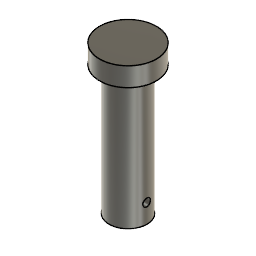
knuckle_joint_assembly (Autodesk Fusion 360 archive; units mm, degrees)
design "pin-knuckle_joint"
part number: 2026-03-14-10-57-53-012
Autodesk Fusion 360 part; units mm, degrees
sketch "Sketch1" plane through (0, 0, 0) normal (0, 0, 1) x (1, 0, 0)
  circle A0 centre (0, 0) radius 22.5
  dimension "d1" = 45
  constraint coincident A0.centre origin
  measures "d1" diameter of A0
extrude "Extrude1" add sketch "Sketch1" against normal blind 15
sketch "Sketch2" plane through (0, 0, -15) normal (0, 0, -1) x (1, 0, 0)
  circle A0 centre (0, 0) radius 22.5
  circle A1 centre (0, 0) radius 15
  dimension "d4" = 30
  constraint coincident A0.centre A1.centre
  measures "d4" diameter of A1
extrude "Extrude2" add sketch "Sketch2" along normal blind 102 contours A1
ref_plane "WorkPlane1" through (-15, 0, 0) normal (1, 0, 0) x (0, 1, 0)
sketch "Sketch5" plane through (-15, 0, 0) normal (1, 0, 0) x (0, 1, 0)
  line L0 (-15, -117) -> (15, -117)
  circle A0 centre (0, -102) radius 3
  dimension "d9" = 6
  measures "d9" diameter of A0
extrude "Extrude3" cut sketch "Sketch5" along normal blind 36

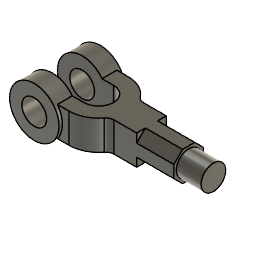
design "fork_sketch"
part number: 2026-03-12-15-10-26-439
Autodesk Fusion 360 part; units mm, degrees
sketch "Sketch7" plane through (0, 0, 0) normal (0, 0, 1) x (1, 0, 0)
  line L0 (31.1769, 18) -> (109, 18)
  line L1 (109, 18) -> (109, -18)
  line L2 (109, -18) -> (31.1769, -18)
  line L3 (0, 0) -> (123.9177, 0)
  line L4 (0, 36) -> (-38, 36)
  line L5 (0, -36) -> (-38, -36)
  line L6 (-38, 36) -> (-38, 18)
  line L7 (-38, -36) -> (-38, -18)
  arc A0 (31.1769, 18) -> (0, 36) centre (0, 0) ccw
  arc A1 (0, -36) -> (31.1769, -18) centre (0, 0) ccw
  arc A2 (0, -18) -> (0, 18) centre (0, 0) ccw
  line L8 (-38, 18) -> (0, 18)
  line L9 (-38, -18) -> (0, -18)
  dimension "d16" = 36
  dimension "d17" = 109
  dimension "d18" = 38
  dimension "d19" = 18
  dimension "d21" = 36
  dimension "d22" = 36
  constraint coincident L3.start A0.centre
  constraint concentric A1 A2
  constraint horizontal L0
  constraint vertical L1
  constraint horizontal L2
  constraint perpendicular L1 L3
  constraint symmetric L0 L2 L3
  constraint tangent L4 A0
  constraint symmetric L3 L4.start L5.start
  constraint symmetric L3 L4.end L5.end
  constraint perpendicular L4 L6
  constraint symmetric L3 L6.end L7.end
  constraint concentric A0 A1
  constraint tangent A2 L8
  constraint tangent A2 L9
  measures "d16" distance of L0.end L1.end
  measures "d17" distance of L3.start L1
  measures "d18" distance of L4.start L4.end
  measures "d19" distance of L4.end L6.end
  measures "d21" diameter of A2
  measures "d22" radius of A0
extrude "Extrude3" add sketch "Sketch7" along normal blind 36
sketch "Sketch8" plane through (0, -18, 0) normal (0, 1, 0) x (-1, 0, 0)
  line L0 (0, 0) -> (38, 0)
  line L1 (38, 0) -> (38, 36)
  line L2 (38, 36) -> (0, 36)
  line L3 (0, 36) -> (0, 0)
  circle A0 centre (38, 18) radius 30
  circle A1 centre (38, 18) radius 15
  dimension "d25" = 60
  dimension "d26" = 30
  constraint midpoint L1 A0.centre
  constraint concentric A0 A1
  measures "d25" diameter of A0
  measures "d26" diameter of A1
extrude "Extrude4" add sketch "Sketch8" against normal blind 22 contours L0 L1 L2 A0 A1 | L0 L1 L2 A0 A1
extrude "Extrude5" cut sketch "Sketch8" against normal blind 40 contours L1 A1 picked at (32.9644, 22.2975)
sketch "Sketch9" plane through (0, 18, 0) normal (0, -1, 0) x (1, 0, 0)
  line L0 (-38, 0) -> (0, 0)
  line L1 (0, 0) -> (0, 36)
  line L2 (0, 36) -> (-38, 36)
  line L3 (-38, 36) -> (-38, 0)
  circle A0 centre (-38, 18) radius 30
  circle A1 centre (-38, 18) radius 15
  dimension "d31" = 60
  dimension "d32" = 30
  constraint midpoint L3 A0.centre
  constraint concentric A0 A1
  measures "d31" diameter of A0
  measures "d32" diameter of A1
extrude "Extrude6" add sketch "Sketch9" against normal blind 22 contours L0 L2 L3 A0 A1 | L0 L2 L3 A0 A1
extrude "Extrude7" cut sketch "Sketch9" against normal blind 26 contours L3 A1 picked at (-35.2114, 22.5991)
sketch "Sketch10" plane through (109, 0, 0) normal (1, 0, 0) x (0, 1, 0)
  line L0 (-18, 0) -> (18, 0)
  line L1 (18, 0) -> (18, 36)
  line L2 (18, 36) -> (-18, 36)
  line L3 (-18, 36) -> (-18, 0)
  line L4 (0, 0) -> (0, 36) construction
  line L5 (-18, 18) -> (18, 18) construction
  line L6 (18, 25.4558) -> (7.4558, 36)
  line L7 (7.4558, 36) -> (-7.4558, 36)
  line L8 (-7.4558, 36) -> (-18, 25.4558)
  line L9 (-18, 25.4558) -> (-18, 10.5442)
  line L10 (-18, 10.5442) -> (-7.4558, 0)
  line L11 (-7.4558, 0) -> (7.4558, 0)
  line L12 (7.4558, 0) -> (18, 10.5442)
  line L13 (18, 10.5442) -> (18, 25.4558)
  point P0 (0, 18)
  constraint coincident L4.start origin
  constraint midpoint L2 L4.end
  constraint midpoint L3 L5.start
  constraint midpoint L1 L5.end
  constraint midpoint L4 P0
extrude "Extrude8" cut sketch "Sketch10" against normal blind 45 contours L1 L2 L6
extrude "Extrude9" cut sketch "Sketch10" against normal blind 45 contours L2 L3 L8
extrude "Extrude10" cut sketch "Sketch10" against normal blind 45 contours L0 L3 L10
extrude "Extrude11" cut sketch "Sketch10" against normal blind 45 contours L0 L1 L12
sketch "Sketch11" plane through (109, 0, 0) normal (1, 0, 0) x (0, 1, 0)
  line L0 (7.4558, 0) -> (18, 10.5442)
  line L1 (18, 10.5442) -> (18, 25.4558)
  line L2 (18, 25.4558) -> (7.4558, 36)
  line L3 (7.4558, 36) -> (-7.4558, 36)
  line L4 (-7.4558, 36) -> (-18, 25.4558)
  line L5 (-18, 25.4558) -> (-18, 10.5442)
  line L6 (-18, 10.5442) -> (-7.4558, 0)
  line L7 (-7.4558, 0) -> (7.4558, 0)
  circle A0 centre (0, 18) radius 15
  dimension "d45" = 30
  measures "d45" diameter of A0
extrude "Extrude12" add sketch "Sketch11" along normal blind 30 contours A0
fillet "Fillet1" radius 10 2 edges at (31.1769, 18, 18) (31.1769, -18, 18)

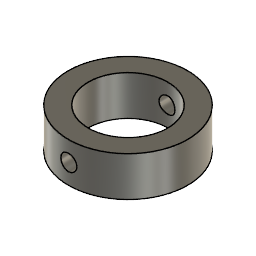
design "COLLAR"
part number: 2026-03-14-12-37-12-628
Autodesk Fusion 360 part; units mm, degrees
sketch "Sketch1" plane through (0, 0, 0) normal (0, 0, 1) x (1, 0, 0)
  circle A0 centre (0, 0) radius 15
  circle A1 centre (0, 0) radius 22.5
  dimension "d1" = 30
  dimension "d2" = 45
  constraint coincident A0.centre A1.centre
  constraint concentric A0 A1
  measures "d1" diameter of A0
  measures "d2" diameter of A1
extrude "Extrude1" add sketch "Sketch1" along normal blind 15
sketch "Sketch2" plane through (0, 0, 0) normal (0, 1, 0) x (1, 0, 0)
ref_plane "WorkPlane1" through (0, -22.5, 0) normal (0, 1, 0) x (0, 0, 1)
sketch "Sketch3" plane through (0, -22.5, 0) normal (0, 1, 0) x (1, 0, 0)
  line L0 (0, 0) -> (0, -15)
  line L1 (-22.5, -15) -> (22.5, -15)
  circle A0 centre (0, -7.5) radius 3
  dimension "d6" = 6
  constraint coincident L0.start origin
  constraint vertical L0
  constraint coincident L0.end L1
  constraint midpoint L0 A0.centre
  measures "d6" diameter of A0
extrude "Extrude2" cut sketch "Sketch3" along normal blind 88

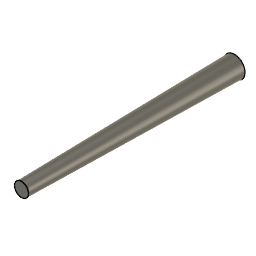
design "taper_pin"
part number: 2026-03-14-12-44-22-029
Autodesk Fusion 360 part; units mm, degrees
sketch "Sketch1" plane through (0, 0, 0) normal (0, 1, 0) x (1, 0, 0)
  circle A0 centre (0, 0) radius 2
  dimension "d1" = 4
  constraint coincident A0.centre origin
  measures "d1" diameter of A0
sketch "Sketch2" plane through (0, 0, 0) normal (0, 1, 0) x (1, 0, 0)
  circle A0 centre (0, 0) radius 2
  dimension "d4" = 4
  constraint coincident A0.centre origin
  measures "d4" diameter of A0
extrude "Extrude2" add sketch "Sketch2" along normal blind 60 draft 0.95
